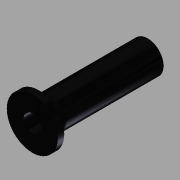
# Autodesk Inventor part: Supporting Plate Standoff Thin
Saved by Autodesk Inventor 2013 (Build 170138000, 138)
## iProperties
Created: 2013-06-26
Part Number: Supporting Plate Standoff Thin
Material: Generic
Document SubType Name: Modeling
Designer: mvarma
Density: 1 g/cm^3
Author: mvarma
Autodesk Inventor part; units mm, degrees
ref_plane "YZ Plane" through (0, 0, 0) normal (1, 0, 0) x (0, 1, 0)
ref_plane "XZ Plane" through (0, 0, 0) normal (0, 1, 0) x (-1, 0, 0)
ref_plane "XY Plane" through (0, 0, 0) normal (0, 0, 1) x (1, 0, 0)
sketch "Sketch1" plane through (0, 0, 0) normal (0, 0, 1) x (1, 0, 0)
  circle A0 centre (0, 0) radius 3.9688
  dimension "d0" = 7.9375
  constraints: 2 coincident, 1 centre point
  measures "d0" diameter of A0
extrude "Extrusion1" add sketch "Sketch1" along normal blind 28.6957
hole "Hole1" at (0, 0, 0) direction (0, 0, 1) diameter 4.318 end through all clearance for "Socket Head Cap Screw" size "#8" standard "Ansi Unified Screw Threads"
sketch "Sketch2" plane through (0, 0, 28.6957) normal (0, 0, 1) x (1, 0, 0)
  circle A0 centre (0, 0) radius 3.9687 projected
  circle A1 centre (0, 0) radius 6.35
  dimension "d10" = 12.7
  constraints: 1 centre point, 1 coincident
  measures "d10" diameter of A1
extrude "Extrusion2" add sketch "Sketch2" against normal blind 1.5875
fillet "Fillet1" radius 3.175 1 edges at (-3.9687, 0, 27.1082)
body "Solid1"
